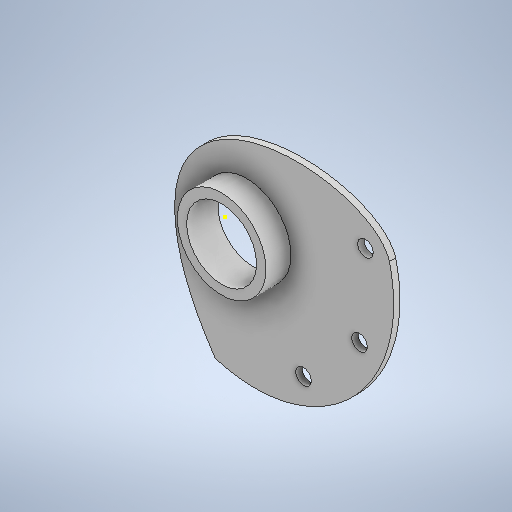
# Autodesk Inventor part: Estructura
Saved by Autodesk Inventor 2025.3 (Build 293356000, 356)
## iProperties
Created: 2025-11-12
Part Number: Estructura
Material: Generic
Document SubType Name: Modeling
Designer: juanm
Density: 1 g/cm^3
Appearance: Default
Author: juanm
Autodesk Inventor part; units mm, degrees
ref_plane "YZ Plane" through (0, 0, 0) normal (1, 0, 0) x (0, 1, 0)
ref_plane "XZ Plane" through (0, 0, 0) normal (0, 1, 0) x (-1, 0, 0)
ref_plane "XY Plane" through (0, 0, 0) normal (0, 0, 1) x (1, 0, 0)
sketch "Sketch1" plane through (0, 0, 0) normal (0, 0, 1) x (1, 0, 0)
  circle A0 centre (25.0838, -31.7051) radius 2.5 projected
  circle A1 centre (43.012, -13.2629) radius 2.5 projected
  circle A2 centre (44.8914, 13.7567) radius 2.5 projected
  circle A3 centre (28.0838, 36.7109) radius 2.5 projected
  circle A4 centre (-0.8935, 43.7288) radius 2.5 projected
  circle A5 centre (-29.5533, 30.4373) radius 2.5 projected
  circle A6 centre (-43.6662, -0.0951) radius 2.5 projected
  circle A7 centre (-47.6662, -52.5951) radius 2.5 projected
  circle A8 centre (-10.6662, -52.5951) radius 2.5 projected
  circle A9 centre (6.8338, -0.0951) radius 4 projected
  line L0 (-3.1662, -60.0951) -> (-3.1662, -40.8213) projected
  spline S0 degree 4 poles (-3.1662, -40.8213) (8.3823, -44.3792) (29.645, -43.1708) (54.7055, -22.2338) (56.6662, 18.5311) (25.1104, 60.0951) (-26.25, 55.8136) (-50.0319, 24.6801) (-51.1662, -0.0951) knots -0.895347 -0.895347 -0.895347 -0.895347 -0.895347 -0.704438 -0.582312 -0.457579 -0.330099 0 0 0 0 0 projected
  line L1 (-51.1662, -0.0951) -> (-56.6662, -60.0951) projected
  line L2 (-56.6662, -60.0951) -> (-3.1662, -60.0951) projected
  circle A10 centre (6.8338, -0.0951) radius 11.2
  line L3 (-3.1662, -40.8213) -> (-29.9162, -34.2051) construction
  line L4 (-29.9162, -34.2051) -> (-46.1662, -23.5051) construction
  line L5 (-46.1662, -23.5051) -> (-51.1662, -0.0951) construction
  spline S1 degree 3 poles (-3.1662, -40.8213) (-29.9162, -34.2051) (-46.1662, -23.5051) (-51.1662, -0.0951) knots 1 1 1 1 2 2 2 2
  point P0 (0, 0)
  dimension "d0" = 22.4
  constraints: 1 centre point, 1 coincident, 3 other
  measures "d0" diameter of A10
extrude "Extrusion1" add sketch "Sketch1" along normal blind 2 contours S1 S0
sketch "Sketch2" plane through (0, 0, 2) normal (0, 0, 1) x (1, 0, 0)
  point P0 (0, 0)
sketch "Sketch3" plane through (0, 0, 2) normal (0, 0, 1) x (1, 0, 0)
  circle A0 centre (6.8338, -0.0951) radius 11.2 projected
  circle A1 centre (6.8338, -0.0951) radius 14.2
  point P0 (0, 0)
  dimension "d3" = 3
  constraints: 1 centre point, 1 coincident
  measures "d3" radial gap between concentric circles of A1 A0
extrude "Extrusion2" add sketch "Sketch3" along normal blind 8
sketch "Sketch4" plane through (0, 0, 2) normal (0, 0, 1) x (1, 0, 0)
  spline S0 degree 4 poles (-3.1662, -40.8213) (-27.2692, -5.9695) (-29.39, 39.4497) (49.0675, 34.0752) (52.786, 13.0688) knots 0 0 0 0 0 1 1 1 1 1
  circle A0 centre (6.8338, -0.0951) radius 14.2 projected
  spline S1 degree 4 poles (-3.1662, -40.8213) (8.3823, -44.3792) (29.645, -43.1708) (54.7055, -22.2338) (56.6662, 18.5311) (25.1104, 60.0951) (-26.25, 55.8136) (-50.0319, 24.6801) (-51.1662, -0.0951) knots 0 0 0 0 0 0.213223 0.349624 0.488937 0.631318 1 1 1 1 1 projected
  spline S2 degree 3 poles (-51.1662, -0.0951) (-46.1662, -23.5051) (-29.9162, -34.2051) (-3.1662, -40.8213) knots 0 0 0 0 1 1 1 1 projected
  circle A1 centre (-43.6662, -0.0951) radius 2.5 projected
  circle A2 centre (-29.5533, 30.4373) radius 2.5 projected
  circle A3 centre (-0.8935, 43.7288) radius 2.5 projected
  circle A4 centre (28.0838, 36.7109) radius 2.5 projected
  circle A5 centre (44.8914, 13.7567) radius 2.5 projected
  circle A6 centre (43.012, -13.2629) radius 2.5 projected
  circle A7 centre (25.0838, -31.7051) radius 2.5 projected
  point P0 (0, 0)
  point P1 (-15.7615, 0.0764)
  point P2 (0.4982, 21.7961)
  point P3 (35.8374, 25.3182)
  point P4 (52.5916, 13.9044)
  constraints: 9 other
extrude "Extrusion3" cut sketch "Sketch4" against normal blind 8 contours S2 S1 S0
body "Solid1"
